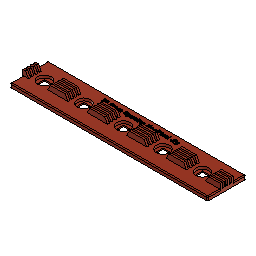
LED_Soldering_Tool (Autodesk Fusion 360 design; units mm, degrees)
Autodesk Fusion 360 part; units mm, degrees
sketch "Body and LED Holes" plane through (0, 0, 0) normal (0, 0, 1) x (1, 0, 0)
  line L0 (-76.25, 29.5) -> (76.25, 29.5)
  line L1 (76.25, 29.5) -> (76.25, 0)
  line L2 (76.25, 0) -> (-76.25, 0)
  line L3 (-76.25, 0) -> (-76.25, 29.5)
  circle A0 centre (-64.5, 14.75) radius 5.1
  line L4 (-64.5, 29.5) -> (-64.5, 0) construction
  line L5 (-67.1, 17.35) -> (-61.9, 17.35)
  line L6 (-61.9, 17.35) -> (-61.9, 12.15)
  line L7 (-61.9, 12.15) -> (-67.1, 12.15)
  line L8 (-67.1, 12.15) -> (-67.1, 17.35)
  line L9 (-61.9, 12.15) -> (-67.1, 17.35) construction
  circle A1 centre (-34, 14.75) radius 5.1
  line L10 (-31.4, 17.35) -> (-31.4, 12.15)
  line L11 (-36.6, 17.35) -> (-31.4, 17.35)
  line L12 (-36.6, 12.15) -> (-36.6, 17.35)
  line L13 (-31.4, 12.15) -> (-36.6, 12.15)
  circle A2 centre (-3.5, 14.75) radius 5.1
  line L14 (-0.9, 17.35) -> (-0.9, 12.15)
  line L15 (-6.1, 17.35) -> (-0.9, 17.35)
  line L16 (-6.1, 12.15) -> (-6.1, 17.35)
  line L17 (-0.9, 12.15) -> (-6.1, 12.15)
  circle A3 centre (27, 14.75) radius 5.1
  line L18 (29.6, 17.35) -> (29.6, 12.15)
  line L19 (24.4, 17.35) -> (29.6, 17.35)
  line L20 (24.4, 12.15) -> (24.4, 17.35)
  line L21 (29.6, 12.15) -> (24.4, 12.15)
  circle A4 centre (57.5, 14.75) radius 5.1
  line L22 (60.1, 17.35) -> (60.1, 12.15)
  line L23 (54.9, 17.35) -> (60.1, 17.35)
  line L24 (54.9, 12.15) -> (54.9, 17.35)
  line L25 (60.1, 12.15) -> (54.9, 12.15)
  dimension "d1" = 152.5
  dimension "d2" = 29.5
  dimension "d3" = 10.2
  dimension "d4" = 11.75
  dimension "d5" = 5.2
  dimension "d6" = 5.2
  dimension "d9" = 30.5
  dimension "d10" = 0
  constraint horizontal L0
  constraint vertical L1
  constraint horizontal L2
  constraint vertical L3
  constraint midpoint origin L2
  constraint coincident L0 L4.start
  constraint coincident L2 L4.end
  constraint perpendicular L2 L4
  constraint midpoint A0.centre L4
  constraint horizontal L5
  constraint vertical L6
  constraint horizontal L7
  constraint vertical L8
  constraint midpoint A0.centre L9
  measures "d1" distance of L0.start L0.end
  measures "d2" distance of L0.start L2.end
  measures "d3" diameter of A0
  measures "d4" distance of L3 L4
  measures "d5" distance of L5.start L5.end
  measures "d6" distance of L5.start L7.end
extrude "Extrude1" add sketch "Body and LED Holes" along normal blind 3 contours L0 L1 L2 L3
extrude "Extrude2" add sketch "Body and LED Holes" along normal blind 1 contours A0 | A1 | A2 | A3 | A4
sketch "Fingers" plane through (0, 0, 3) normal (0, 0, 1) x (-1, 0, 0)
  circle A0 centre (64.5, -14.75) radius 5.1
  circle A1 centre (-57.5, -14.75) radius 5.1
  circle A2 centre (-27, -14.75) radius 5.1
  circle A3 centre (3.5, -14.75) radius 5.1
  circle A4 centre (34, -14.75) radius 5.1
  line L0 (76.25, 0) -> (-76.25, 0)
  line L1 (-76.25, 0) -> (-76.25, -29.5)
  line L2 (-76.25, -29.5) -> (76.25, -29.5)
  line L3 (76.25, -29.5) -> (76.25, 0)
  line L4 (-3.88, -19.7) -> (-19.62, -19.7)
  line L5 (-19.62, -19.7) -> (-19.62, -18.2)
  line L6 (-19.62, -18.2) -> (-3.88, -18.2)
  line L7 (-3.88, -18.2) -> (-3.88, -19.7)
  line L8 (-3.88, -16.9) -> (-19.62, -16.9)
  line L9 (-19.62, -16.9) -> (-19.62, -15.4)
  line L10 (-19.62, -15.4) -> (-3.88, -15.4)
  line L11 (-3.88, -15.4) -> (-3.88, -16.9)
  line L12 (-3.88, -14.1) -> (-19.62, -14.1)
  line L13 (-19.62, -14.1) -> (-19.62, -12.6)
  line L14 (-19.62, -12.6) -> (-3.88, -12.6)
  line L15 (-3.88, -12.6) -> (-3.88, -14.1)
  line L16 (-3.88, -11.3) -> (-19.62, -11.3)
  line L17 (-19.62, -11.3) -> (-19.62, -9.8)
  line L18 (-19.62, -9.8) -> (-3.88, -9.8)
  line L19 (-3.88, -9.8) -> (-3.88, -11.3)
  line L20 (-3.88, -15.4) -> (-19.62, -14.1) construction
  line L21 (8.6, -14.75) -> (-32.1, -14.75) construction
  line L22 (-64.88, -15.4) -> (-80.62, -14.1) construction
  line L23 (-80.62, -9.8) -> (-64.88, -9.8)
  line L24 (-64.88, -14.1) -> (-80.62, -14.1)
  line L25 (-80.62, -14.1) -> (-80.62, -12.6)
  line L26 (-64.88, -12.6) -> (-64.88, -14.1)
  line L27 (-80.62, -11.3) -> (-80.62, -9.8)
  line L28 (-64.88, -11.3) -> (-80.62, -11.3)
  line L29 (-80.62, -16.9) -> (-80.62, -15.4)
  line L30 (-64.88, -15.4) -> (-64.88, -16.9)
  line L31 (-64.88, -16.9) -> (-80.62, -16.9)
  line L32 (-80.62, -15.4) -> (-64.88, -15.4)
  line L33 (-80.62, -12.6) -> (-64.88, -12.6)
  line L34 (-64.88, -19.7) -> (-80.62, -19.7)
  line L35 (-80.62, -19.7) -> (-80.62, -18.2)
  line L36 (-64.88, -18.2) -> (-64.88, -19.7)
  line L37 (-80.62, -18.2) -> (-64.88, -18.2)
  line L38 (-64.88, -9.8) -> (-64.88, -11.3)
  line L39 (-34.38, -15.4) -> (-50.12, -14.1) construction
  line L40 (-50.12, -9.8) -> (-34.38, -9.8)
  line L41 (-34.38, -14.1) -> (-50.12, -14.1)
  line L42 (-50.12, -14.1) -> (-50.12, -12.6)
  line L43 (-34.38, -12.6) -> (-34.38, -14.1)
  line L44 (-50.12, -11.3) -> (-50.12, -9.8)
  line L45 (-34.38, -11.3) -> (-50.12, -11.3)
  line L46 (-50.12, -16.9) -> (-50.12, -15.4)
  line L47 (-34.38, -15.4) -> (-34.38, -16.9)
  line L48 (-34.38, -16.9) -> (-50.12, -16.9)
  line L49 (-50.12, -15.4) -> (-34.38, -15.4)
  line L50 (-50.12, -12.6) -> (-34.38, -12.6)
  line L51 (-34.38, -19.7) -> (-50.12, -19.7)
  line L52 (-50.12, -19.7) -> (-50.12, -18.2)
  line L53 (-34.38, -18.2) -> (-34.38, -19.7)
  line L54 (-50.12, -18.2) -> (-34.38, -18.2)
  line L55 (-34.38, -9.8) -> (-34.38, -11.3)
  line L56 (26.62, -15.4) -> (10.88, -14.1) construction
  line L57 (10.88, -9.8) -> (26.62, -9.8)
  line L58 (26.62, -14.1) -> (10.88, -14.1)
  line L59 (10.88, -14.1) -> (10.88, -12.6)
  line L60 (26.62, -12.6) -> (26.62, -14.1)
  line L61 (10.88, -11.3) -> (10.88, -9.8)
  line L62 (26.62, -11.3) -> (10.88, -11.3)
  line L63 (10.88, -16.9) -> (10.88, -15.4)
  line L64 (26.62, -15.4) -> (26.62, -16.9)
  line L65 (26.62, -16.9) -> (10.88, -16.9)
  line L66 (10.88, -15.4) -> (26.62, -15.4)
  line L67 (10.88, -12.6) -> (26.62, -12.6)
  line L68 (26.62, -19.7) -> (10.88, -19.7)
  line L69 (10.88, -19.7) -> (10.88, -18.2)
  line L70 (26.62, -18.2) -> (26.62, -19.7)
  line L71 (10.88, -18.2) -> (26.62, -18.2)
  line L72 (26.62, -9.8) -> (26.62, -11.3)
  line L73 (57.12, -15.4) -> (41.38, -14.1) construction
  line L74 (41.38, -9.8) -> (57.12, -9.8)
  line L75 (57.12, -14.1) -> (41.38, -14.1)
  line L76 (41.38, -14.1) -> (41.38, -12.6)
  line L77 (57.12, -12.6) -> (57.12, -14.1)
  line L78 (41.38, -11.3) -> (41.38, -9.8)
  line L79 (57.12, -11.3) -> (41.38, -11.3)
  line L80 (41.38, -16.9) -> (41.38, -15.4)
  line L81 (57.12, -15.4) -> (57.12, -16.9)
  line L82 (57.12, -16.9) -> (41.38, -16.9)
  line L83 (41.38, -15.4) -> (57.12, -15.4)
  line L84 (41.38, -12.6) -> (57.12, -12.6)
  line L85 (57.12, -19.7) -> (41.38, -19.7)
  line L86 (41.38, -19.7) -> (41.38, -18.2)
  line L87 (57.12, -18.2) -> (57.12, -19.7)
  line L88 (41.38, -18.2) -> (57.12, -18.2)
  line L89 (57.12, -9.8) -> (57.12, -11.3)
  line L90 (87.62, -15.4) -> (71.88, -14.1) construction
  line L91 (71.88, -9.8) -> (87.62, -9.8)
  line L92 (87.62, -14.1) -> (71.88, -14.1)
  line L93 (71.88, -14.1) -> (71.88, -12.6)
  line L94 (87.62, -12.6) -> (87.62, -14.1)
  line L95 (71.88, -11.3) -> (71.88, -9.8)
  line L96 (87.62, -11.3) -> (71.88, -11.3)
  line L97 (71.88, -16.9) -> (71.88, -15.4)
  line L98 (87.62, -15.4) -> (87.62, -16.9)
  line L99 (87.62, -16.9) -> (71.88, -16.9)
  line L100 (71.88, -15.4) -> (87.62, -15.4)
  line L101 (71.88, -12.6) -> (87.62, -12.6)
  line L102 (87.62, -19.7) -> (71.88, -19.7)
  line L103 (71.88, -19.7) -> (71.88, -18.2)
  line L104 (87.62, -18.2) -> (87.62, -19.7)
  line L105 (71.88, -18.2) -> (87.62, -18.2)
  line L106 (87.62, -9.8) -> (87.62, -11.3)
  dimension "d15" = 15.74
  dimension "d16" = 1.5
  dimension "d19" = 0
  dimension "d20" = 2.8
  dimension "d23" = 30.5
  dimension "d24" = 0
  constraint horizontal L4
  constraint vertical L5
  constraint horizontal L6
  constraint vertical L7
  constraint coincident A3 L21.start
  constraint coincident A2 L21.end
  constraint coincident A2.centre L21
  constraint coincident A3.centre L21
  constraint midpoint L20 L21
  measures "d15" distance of L4.start L4.end
  measures "d16" distance of L4.start L6.end
extrude "Extrude3" add sketch "Fingers" along normal blind 4 contours L3 L91 L95 L96 | L1 L23 L28 L38 | L3 L92 L93 L101 | L1 L24 L26 L33 | L3 L97 L99 L100 | L1 L30 L31 L32 | L3 L102 L103 L105 | L1 L34 L36 L37 | L4 L5 L6 L7 | L8 L9 L10 L11 | L12 L13 L14 L15 | L16 L17 L18 L19 | L40 L44 L45 L55 | L41 L42 L43 L50 | L46 L47 L48 L49 | L51 L52 L53 L54 | L57 L61 L62 L72 | L58 L59 L60 L67 | L63 L64 L65 L66 | L68 L69 L70 L71 | L74 L78 L79 L89 | L75 L76 L77 L84 | L80 L81 L82 L83 | L85 L86 L87 L88
chamfer "Chamfer1" distance 2.3 angle 60 40 edges at (-10.88, 13.35, 7) (-10.88, 16.15, 7) (-10.88, 18.95, 7) (-26.62, 18.95, 7) (-26.62, 16.15, 7) (-26.62, 13.35, 7) (-10.88, 10.55, 7) (-26.62, 10.55, 7) (-41.38, 10.55, 7) (-41.38, 13.35, 7) (-41.38, 16.15, 7) (-41.38, 18.95, 7) (-57.12, 18.95, 7) (-57.12, 16.15, 7) (-57.12, 13.35, 7) (-57.12, 10.55, 7) (-71.88, 10.55, 7) (-71.88, 13.35, 7) (-71.88, 16.15, 7) (-71.88, 18.95, 7) (3.88, 10.55, 7) (3.88, 13.35, 7) (3.88, 16.15, 7) (3.88, 18.95, 7) (19.62, 10.55, 7) (19.62, 13.35, 7) (19.62, 16.15, 7) (19.62, 18.95, 7) (34.38, 10.55, 7) (34.38, 13.35, 7) (34.38, 16.15, 7) (34.38, 18.95, 7) (50.12, 18.95, 7) (50.12, 16.15, 7) (50.12, 13.35, 7) (50.12, 10.55, 7) (64.88, 10.55, 7) (64.88, 13.35, 7) (64.88, 16.15, 7) (64.88, 18.95, 7) measured on face at (-21.3733, 13.6, 7) measured on face at (-16.1267, 15.9, 7) measured on face at (-21.3733, 19.2, 7) measured on face at (-21.3733, 19.2, 7) measured on face at (-16.1267, 15.9, 7) measured on face at (-21.3733, 13.6, 7) measured on face at (-16.1267, 10.3, 7) measured on face at (-16.1267, 10.3, 7) measured on face at (-51.8733, 10.8, 7) measured on face at (-51.8733, 13.6, 7) measured on face at (-46.6267, 15.9, 7) measured on face at (-51.8733, 19.2, 7) measured on face at (-51.8733, 19.2, 7) measured on face at (-46.6267, 15.9, 7) measured on face at (-51.8733, 13.6, 7) measured on face at (-51.8733, 10.8, 7) measured on face at (-73.3367, 10.3, 7) measured on face at (-73.3367, 13.1, 7) measured on face at (-74.7933, 15.9, 7) measured on face at (-73.3367, 18.7, 7) measured on face at (14.3733, 10.8, 7) measured on face at (14.3733, 13.6, 7) measured on face at (14.3733, 16.4, 7) measured on face at (14.3733, 19.2, 7) measured on face at (14.3733, 10.8, 7) measured on face at (14.3733, 13.6, 7) measured on face at (14.3733, 16.4, 7) measured on face at (14.3733, 19.2, 7) measured on face at (44.8733, 10.3, 7) measured on face at (39.6267, 13.6, 7) measured on face at (44.8733, 15.9, 7) measured on face at (39.6267, 19.2, 7) measured on face at (39.6267, 19.2, 7) measured on face at (44.8733, 15.9, 7) measured on face at (39.6267, 13.6, 7) measured on face at (44.8733, 10.3, 7) measured on face at (72.46, 10.3, 7) measured on face at (72.46, 13.1, 7) measured on face at (68.67, 16.4, 7) measured on face at (72.46, 18.7, 7)
sketch "Text" plane through (0, 0, 3) normal (0, 0, 1) x (-1, 0, 0)
  line L0 (-64.88, -11.3) -> (-76.25, -11.3)
  line L1 (-76.25, -11.3) -> (-76.25, -12.6)
  line L2 (-76.25, -12.6) -> (-64.88, -12.6)
  line L3 (-64.88, -12.6) -> (-64.88, -14.1)
  line L4 (-64.88, -14.1) -> (-76.25, -14.1)
  line L5 (-76.25, -14.1) -> (-76.25, -15.4)
  line L6 (-76.25, -15.4) -> (-64.88, -15.4)
  line L7 (-64.88, -15.4) -> (-64.88, -16.9)
  line L8 (-64.88, -16.9) -> (-76.25, -16.9)
  line L9 (-76.25, -16.9) -> (-76.25, -18.2)
  line L10 (-76.25, -18.2) -> (-64.88, -18.2)
  line L11 (-64.88, -18.2) -> (-64.88, -19.7)
  line L12 (-64.88, -19.7) -> (-76.25, -19.7)
  line L13 (-76.25, -19.7) -> (-76.25, -29.5)
  line L14 (-76.25, -29.5) -> (76.25, -29.5)
  line L15 (76.25, -29.5) -> (76.25, -19.7)
  line L16 (76.25, -19.7) -> (71.88, -19.7)
  line L17 (71.88, -19.7) -> (71.88, -18.2)
  line L18 (71.88, -18.2) -> (76.25, -18.2)
  line L19 (76.25, -18.2) -> (76.25, -16.9)
  line L20 (76.25, -16.9) -> (71.88, -16.9)
  line L21 (71.88, -16.9) -> (71.88, -15.4)
  line L22 (71.88, -15.4) -> (76.25, -15.4)
  line L23 (76.25, -15.4) -> (76.25, -14.1)
  line L24 (76.25, -14.1) -> (71.88, -14.1)
  line L25 (71.88, -14.1) -> (71.88, -12.6)
  line L26 (71.88, -12.6) -> (76.25, -12.6)
  line L27 (76.25, -12.6) -> (76.25, -11.3)
  line L28 (76.25, -11.3) -> (71.88, -11.3)
  line L29 (71.88, -11.3) -> (71.88, -9.8)
  line L30 (71.88, -9.8) -> (76.25, -9.8)
  line L31 (76.25, -9.8) -> (76.25, 0)
  line L32 (76.25, 0) -> (-76.25, 0)
  line L33 (-76.25, 0) -> (-76.25, -9.8)
  line L34 (-76.25, -9.8) -> (-64.88, -9.8)
  line L35 (-64.88, -9.8) -> (-64.88, -11.3)
  line L36 (-34.38, -9.8) -> (-34.38, -11.3)
  line L37 (-34.38, -11.3) -> (-50.12, -11.3)
  line L38 (-50.12, -11.3) -> (-50.12, -9.8)
  line L39 (-50.12, -9.8) -> (-34.38, -9.8)
  line L40 (-3.88, -18.2) -> (-3.88, -19.7)
  line L41 (-3.88, -19.7) -> (-19.62, -19.7)
  line L42 (-19.62, -19.7) -> (-19.62, -18.2)
  line L43 (-19.62, -18.2) -> (-3.88, -18.2)
  line L44 (26.62, -9.8) -> (26.62, -11.3)
  line L45 (26.62, -11.3) -> (10.88, -11.3)
  line L46 (10.88, -11.3) -> (10.88, -9.8)
  line L47 (10.88, -9.8) -> (26.62, -9.8)
  line L48 (41.38, -18.2) -> (57.12, -18.2)
  line L49 (57.12, -18.2) -> (57.12, -19.7)
  line L50 (57.12, -19.7) -> (41.38, -19.7)
  line L51 (41.38, -19.7) -> (41.38, -18.2)
  line L52 (57.12, -9.8) -> (57.12, -11.3)
  line L53 (57.12, -11.3) -> (41.38, -11.3)
  line L54 (41.38, -11.3) -> (41.38, -9.8)
  line L55 (41.38, -9.8) -> (57.12, -9.8)
  line L56 (10.88, -18.2) -> (26.62, -18.2)
  line L57 (26.62, -18.2) -> (26.62, -19.7)
  line L58 (26.62, -19.7) -> (10.88, -19.7)
  line L59 (10.88, -19.7) -> (10.88, -18.2)
  line L60 (-3.88, -9.8) -> (-3.88, -11.3)
  line L61 (-3.88, -11.3) -> (-19.62, -11.3)
  line L62 (-19.62, -11.3) -> (-19.62, -9.8)
  line L63 (-19.62, -9.8) -> (-3.88, -9.8)
  line L64 (-50.12, -18.2) -> (-34.38, -18.2)
  line L65 (-34.38, -18.2) -> (-34.38, -19.7)
  line L66 (-34.38, -19.7) -> (-50.12, -19.7)
  line L67 (-50.12, -19.7) -> (-50.12, -18.2)
  line L68 (-50.12, -12.6) -> (-34.38, -12.6)
  line L69 (-34.38, -12.6) -> (-34.38, -14.1)
  line L70 (-34.38, -14.1) -> (-50.12, -14.1)
  line L71 (-50.12, -14.1) -> (-50.12, -12.6)
  line L72 (-3.88, -15.4) -> (-3.88, -16.9)
  line L73 (-3.88, -16.9) -> (-19.62, -16.9)
  line L74 (-19.62, -16.9) -> (-19.62, -15.4)
  line L75 (-19.62, -15.4) -> (-3.88, -15.4)
  line L76 (10.88, -12.6) -> (26.62, -12.6)
  line L77 (26.62, -12.6) -> (26.62, -14.1)
  line L78 (26.62, -14.1) -> (10.88, -14.1)
  line L79 (10.88, -14.1) -> (10.88, -12.6)
  line L80 (41.38, -15.4) -> (57.12, -15.4)
  line L81 (57.12, -15.4) -> (57.12, -16.9)
  line L82 (57.12, -16.9) -> (41.38, -16.9)
  line L83 (41.38, -16.9) -> (41.38, -15.4)
  line L84 (41.38, -12.6) -> (57.12, -12.6)
  line L85 (57.12, -12.6) -> (57.12, -14.1)
  line L86 (57.12, -14.1) -> (41.38, -14.1)
  line L87 (41.38, -14.1) -> (41.38, -12.6)
  line L88 (10.88, -15.4) -> (26.62, -15.4)
  line L89 (26.62, -15.4) -> (26.62, -16.9)
  line L90 (26.62, -16.9) -> (10.88, -16.9)
  line L91 (10.88, -16.9) -> (10.88, -15.4)
  line L92 (-3.88, -12.6) -> (-3.88, -14.1)
  line L93 (-3.88, -14.1) -> (-19.62, -14.1)
  line L94 (-19.62, -14.1) -> (-19.62, -12.6)
  line L95 (-19.62, -12.6) -> (-3.88, -12.6)
  line L96 (-50.12, -15.4) -> (-34.38, -15.4)
  line L97 (-34.38, -15.4) -> (-34.38, -16.9)
  line L98 (-34.38, -16.9) -> (-50.12, -16.9)
  line L99 (-50.12, -16.9) -> (-50.12, -15.4)
  circle A0 centre (64.5, -14.75) radius 5.1
  circle A1 centre (-57.5, -14.75) radius 5.1
  circle A2 centre (-27, -14.75) radius 5.1
  circle A3 centre (3.5, -14.75) radius 5.1
  circle A4 centre (34, -14.75) radius 5.1
  line L100 (76.25, -19.7) -> (-76.25, -19.7) construction
  line L101 (0, -19.7) -> (0, -29.5) construction
  line L102 (76.25, -19.7) -> (-76.25, -19.7) construction
  line L103 (-76.25, -19.7) -> (-76.25, -29.5) construction
  line L104 (-76.25, -29.5) -> (76.25, -29.5) construction
  line L105 (76.25, -29.5) -> (76.25, -19.7) construction
  dimension "d29" = 3
  text T0 "30.5mm Spacing NeoPixel Jig" font "Arial" height 3 bold align centre middle in box 152.5 x 9.8 at (76.25, -19.7) x (-1, 0) y (0, -1) spacing 1
  constraint coincident L15 L16.start
  constraint coincident L13 L12.end
  constraint perpendicular L13 L100
  constraint collinear L41 L100
  constraint midpoint L100 L101.start
  constraint midpoint L14 L101.end
  constraint midpoint L14 L104
  constraint collinear L100 L102
  constraint collinear L13 L103
extrude "Extrude4" cut sketch "Text" against normal blind 1 text T0
fillet "Fillet1" radius 0.75 10 edges at (-76.25, 0, 1.5) (0, 0, 3) (-76.25, 4.9, 3) (-76.25, 24.6, 3) (-76.25, 29.5, 1.5) (0, 29.5, 3) (76.25, 0, 1.5) (76.25, 4.9, 3) (76.25, 24.6, 3) (76.25, 29.5, 1.5)
named bodies: "Soldering Tool"
